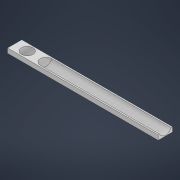
# Autodesk Inventor part: Trilho 60 minutos
Saved by Autodesk Inventor 2022 (Build 260153000, 153)
## iProperties
Created: 2023-05-09
Part Number: Trilho 60 minutos
Material: Genérico
Document SubType Name: Modeling
Designer: jpjoa
Density: 1 g/cm^3
Appearance: Padrão
Author: jpjoa
Autodesk Inventor part; units mm, degrees
ref_plane "YZ Plane" through (0, 0, 0) normal (1, 0, 0) x (0, 1, 0)
ref_plane "XZ Plane" through (0, 0, 0) normal (0, 1, 0) x (-1, 0, 0)
ref_plane "XY Plane" through (0, 0, 0) normal (0, 0, 1) x (1, 0, 0)
sketch "Esboço2" plane through (0, 0, 0) normal (0, 1, 0) x (-1, 0, 0)
  line L0 (0, 0) -> (-216, 0)
  line L1 (-216, 0) -> (-216, -20.4)
  line L2 (-216, -20.4) -> (0, -20.4)
  line L3 (0, -20.4) -> (0, 0)
  circle A0 centre (-18, -10.2) radius 9
  line L4 (-36, -19.2) -> (-216, -19.2)
  line L5 (-36, -19.2) -> (-36, -1.2)
  line L6 (-216, -1.2) -> (-36, -1.2)
  point P0 (0, -10.2)
  dimension "d5" = 216
  dimension "d6" = 20.4
  dimension "d7" = 18
  dimension "d8" = 1.2
  dimension "d9" = 36
  dimension "d10" = 18
  dimension "d11" = 1.2
  constraints: 14 end point, 4 perpendicular, 2 point on line, 1 centre point, 1 horizontal, 1 horizontal alignment, 1 midpoint, 1 parallel, 1 vertical
  measures "d5" distance of L0.start L0.end
  measures "d6" distance of L0.end L1.end
  measures "d7" diameter of A0
  measures "d8" distance between parallel lines of L2 L4
  measures "d9" distance between parallel lines of L3 L5
  measures "d10" distance from line of L3 A0.centre
  measures "d11" distance between parallel lines of L0 L6
extrude "Extrusão1" add sketch "Esboço2" against normal blind 1.2 contours L3 L2 L1 L4 L5 L6 L0 | L6 L5 L4 L1 | A0
extrude "Extrusão2" add sketch "Esboço2" along normal blind 9 contours L3 L2 L1 L4 L5 L6 L0
fillet "Arredondamento2" radius 9 3 edges at (27, 0, -10.2) (126, 0, -19.2) (126, 0, -1.2)
fillet "Arredondamento3" radius 9 5 edges at (36, 8.9999, -19.2) (36, 2.636, -16.564) (36, 0, -10.2) (36, 2.636, -3.836) (36, 8.9999, -1.2)
sketch "Esboço3" plane through (0, -1.2, 0) normal (0, 0, 1) x (1, 0, 0)
  line L0 (216, 1.2) -> (216, 0)
  line L1 (0, 6.6) -> (216, 6.6)
  line L2 (216, 6.6) -> (216, 1.2)
  line L3 (216, 10.2) -> (216, 0) projected
  line L4 (0, 6.6) -> (0, 10.2)
  line L5 (0, 10.2) -> (216, 10.2) projected
  line L6 (0, 10.2) -> (216, 10.2)
  line L7 (216, 10.2) -> (216, 6.6)
  line L8 (0, 0) -> (0, 10.2) projected
  point P0 (216, 3.9)
  point P1 (216, 5.1)
  point P2 (216, 0.6)
  point P3 (216, 5.1)
  point P4 (0, 8.4)
  point P5 (0, 5.1)
  dimension "d20" = 1.2
  dimension "d21" = 5.4
  constraints: 12 end point, 6 midpoint, 3 vertical alignment, 2 perpendicular, 1 coincident, 1 collinear, 1 parallel
  measures "d20" distance of L0.start L0.end
  measures "d21" distance of L1.end L0.start
extrude "Extrusão3" cut sketch "Esboço3" against normal through all
equation "\"d5\" = 12 * Diâmetro_esfera"
equation "\"d6\" = Diâmetro_esfera + 2 * Margem"
equation "\"d7\" = Diâmetro_esfera"
equation "\"d8\" = Margem"
equation "\"d9\" = 2 * Diâmetro_esfera"
equation "\"d10\" = Diâmetro_esfera"
equation "\"d11\" = Margem"
equation "\"d13\" = Margem"
equation "\"d15\" = 0.5 * Diâmetro_esfera"
equation "\"d18\" = 0.5 * Diâmetro_esfera"
equation "\"d19\" = 0.5 * Diâmetro_esfera"
equation "\"d20\" = Margem"
equation "\"d21\" = 0.3 * Diâmetro_esfera"
equation "\"Diâmetro_esfera\" = 18"
equation "\"Margem\" = 3 * Filamento"
equation "\"Filamento\" = 0.4"
